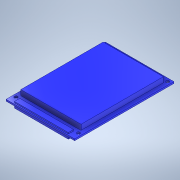
# Autodesk Inventor part: Ecran
Saved by Autodesk Inventor 2020 (Build 240168000, 168)
## iProperties
Created: 2020-01-01
Part Number: Ecran
Material: Argent
Document SubType Name: Modeling
Designer: Manuel Enzo
Density: 10.49 g/cm^3
Appearance: Bleu - Peinture murale - Brillant
Author: Manuel Enzo
Autodesk Inventor part; units mm, degrees
ref_plane "YZ Plane" through (0, 0, 0) normal (1, 0, 0) x (0, 1, 0)
ref_plane "XZ Plane" through (0, 0, 0) normal (0, 1, 0) x (-1, 0, 0)
ref_plane "XY Plane" through (0, 0, 0) normal (0, 0, 1) x (1, 0, 0)
sketch "Esquisse1" plane through (0, 0, 0) normal (0, 1, 0) x (-1, 0, 0)
  line L0 (0, 0) -> (65, 0)
  line L1 (65, 0) -> (65, -94)
  line L2 (65, -94) -> (0, -94)
  line L3 (0, -94) -> (0, 0)
  line L4 (61, -88) -> (4, -88)
  line L5 (4, -88) -> (4, -10)
  line L6 (4, -10) -> (61, -10)
  line L7 (61, -10) -> (61, -88)
  circle A0 centre (62, -91) radius 2.5
  circle A1 centre (62, -91) radius 1.5
  circle A2 centre (3, -91) radius 2.5
  circle A3 centre (3, -91) radius 1.5
  circle A4 centre (3, -6.5) radius 2.5
  circle A5 centre (3, -6.5) radius 1.5
  circle A6 centre (62, -6.5) radius 2.5
  circle A7 centre (62, -6.5) radius 1.5
  dimension "d0" = 65
  dimension "d1" = 94
  dimension "d2" = 4
  dimension "d3" = 4
  dimension "d4" = 6
  dimension "d5" = 10
  dimension "d6" = 3
  dimension "d7" = 5
  dimension "d8" = 3
  dimension "d9" = 1
  dimension "d10" = 1
  dimension "d11" = 3
  dimension "d12" = 3
  dimension "d13" = 5
  dimension "d14" = 1
  dimension "d15" = 5
  dimension "d16" = 3
  dimension "d17" = 3.5
  dimension "d18" = 6.5
  dimension "d19" = 1
  dimension "d20" = 3
  dimension "d21" = 3.5
  dimension "d22" = 5
  dimension "d23" = 6.5
  constraints: 16 end point, 8 centre point, 4 coincident, 4 parallel, 2 horizontal, 2 perpendicular
  measures "d0" distance between parallel lines of L1 L3
  measures "d1" distance between parallel lines of L0 L2
  measures "d2" distance between parallel lines of L1 L7
  measures "d3" distance between parallel lines of L3 L5
  measures "d4" distance between parallel lines of L2 L4
  measures "d5" distance between parallel lines of L0 L6
  measures "d6" distance from line of L1 A0.centre
  measures "d7" diameter of A0
  measures "d8" distance from line of L2 A0.centre
  measures "d9" radial gap between concentric circles of A0 A1
  measures "d10" radial gap between concentric circles of A2 A3
  measures "d11" distance from line of L3 A2.centre
  measures "d12" distance from line of L2 A2.centre
  measures "d13" diameter of A2
  measures "d14" radial gap between concentric circles of A4 A5
  measures "d15" diameter of A4
  measures "d16" distance from line of L3 A4.centre
  measures "d17" distance from line of L6 A4.centre
  measures "d18" distance from line of L0 A4.centre
  measures "d19" radial gap between concentric circles of A6 A7
  measures "d20" distance from line of L1 A6.centre
  measures "d21" distance from line of L6 A6.centre
  measures "d22" diameter of A6
  measures "d23" distance from line of L0 A6.centre
extrude "Extrusion2" add sketch "Esquisse1" along normal blind 1.5 contours L0 L1 L2 L3 | L4 L5 L6 L7
extrude "Extrusion4" add sketch "Esquisse1" along normal blind 6.5 contours L4 L5 L6 L7
extrude "Extrusion5" add sketch "Esquisse1" along normal blind 1.5 contours A0 | A2 | A4 | A6
sketch "Esquisse4" plane through (0, 0, 0) normal (0, -1, 0) x (1, 0, 0)
  line L0 (-7, -1) -> (-58, -1)
  line L1 (-58, -1) -> (-58, -6)
  line L2 (-58, -6) -> (-7, -6)
  line L3 (-7, -6) -> (-7, -1)
  line L4 (-65, 0) -> (0, 0) projected
  line L5 (0, 0) -> (0, -94) projected
  line L6 (-65, -94) -> (-65, 0) projected
  dimension "d69" = 1
  dimension "d70" = 51
  dimension "d71" = 5
  dimension "d72" = 7
  dimension "d73" = 7
  constraints: 8 end point, 2 parallel, 1 horizontal, 1 perpendicular
  measures "d69" distance between parallel lines of L4 L0
  measures "d70" distance of L1.end L2.end
  measures "d71" distance between parallel lines of L0 L2
  measures "d72" distance between parallel lines of L5 L3
  measures "d73" distance between parallel lines of L6 L1
extrude "Extrusion6" add sketch "Esquisse4" along normal blind 2.75
extrude "Extrusion7" add sketch "Esquisse4" against normal blind 2.75
